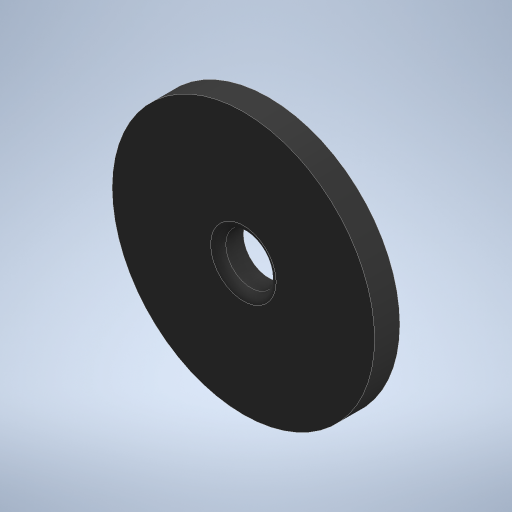
# Autodesk Inventor part: Rubber
Saved by Autodesk Inventor 2024 (Build 280153000, 153)
## iProperties
Created: 2024-03-23
Part Number: Rubber
Material: Generic
Document SubType Name: Modeling
Designer: MSI-C
Density: 1 g/cm^3
Appearance: Rubber - Black
Mass: 10.2259 g
Surface Area: 50.6425 cm^2
Volume: 10.2259 cm^3
Author: MSI-C
Autodesk Inventor part; units mm, degrees
ref_plane "YZ Plane" through (0, 0, 0) normal (1, 0, 0) x (0, 1, 0)
ref_plane "XZ Plane" through (0, 0, 0) normal (0, 1, 0) x (-1, 0, 0)
ref_plane "XY Plane" through (0, 0, 0) normal (0, 0, 1) x (1, 0, 0)
sketch "Sketch1" plane through (0, 0, 0) normal (0, 0, 1) x (1, 0, 0)
  circle A0 centre (0, 0) radius 26
  circle A1 centre (0, 0) radius 5
  dimension "d0" = 52
  dimension "d1" = 10
  constraints: 2 centre point, 2 coincident
  measures "d0" diameter of A0
  measures "d1" diameter of A1
extrude "Extrusion1" add sketch "Sketch1" along normal mid plane 5
fillet "Fillet1" radius 1.5 1 edges at (-5, 0, 2.5)
body "Solid1"
